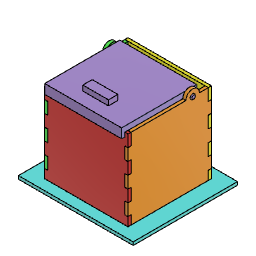
box (Autodesk Fusion 360 design; units mm, degrees)
Autodesk Fusion 360 part; units mm, degrees
note: some values were not read from the file. Set by a fixed rule: which sketch regions a step uses.
sketch "Sketch2" plane through (0, 0, 0) normal (0, 1, 0) x (1, 0, 0)
  line L0 (0, 0) -> (80, 0)
  line L1 (80, 0) -> (80, -80)
  line L2 (80, -80) -> (0, -80)
  line L3 (0, -80) -> (0, 0)
  dimension "d65" = 80
  dimension "d66" = 80
  constraint horizontal L0
  constraint vertical L1
  constraint horizontal L2
  constraint vertical L3
  constraint coincident L0.start L3.end
  measures "d65" distance of L0.start L0.end
  measures "d66" distance of L0.start L2.end
extrude "Extrude1" add sketch "Sketch2" along normal blind 3 makes body 1 in component "Front"
sketch "Sketch1" plane through (0, 0, 0) normal (0, -1, 0) x (1, 0, 0) in component "Front"
  line L0 (80, 80) -> (0, 80)
  line L1 (0, 80) -> (0, 0)
  line L2 (0, 0) -> (80, 0)
  line L3 (80, 0) -> (80, 80)
  line L4 (7.2727, 0) -> (14.5455, 0)
  line L5 (14.5455, 0) -> (14.5455, 3)
  line L6 (14.5455, 3) -> (7.2727, 3)
  line L7 (7.2727, 3) -> (7.2727, 0)
  dimension "d69" = 7.2727
  dimension "d70" = 7.2727
  dimension "d71" = 3
  constraint horizontal L4
  constraint vertical L5
  constraint horizontal L6
  constraint vertical L7
  constraint coincident L2 L4.start
  measures "d69" distance of L5.end L6.end
  measures "d70" distance of L1 L7
  measures "d71" distance of L4 L6
extrude "Extrude2" cut sketch "Sketch1" against normal blind 3 contours L2 L4 L5 L6 L7 bodies 1 in component "Front"
pattern_linear "R-Pattern1" count 5 spacing 14.5455 along (1, 0, 0) of "Extrude2" in component "Front"
sketch "Sketch2 (2)" plane through (80, 0, 0) normal (1, 0, 0) x (0, 1, 0) in component "Front"
  line L0 (0, 80) -> (0, 0)
  line L1 (0, 0) -> (3, 0)
  line L2 (3, 0) -> (3, 80)
  line L3 (3, 80) -> (0, 80)
  line L4 (0, 22.8571) -> (3, 22.8571)
  line L5 (3, 22.8571) -> (3, 11.4286)
  line L6 (3, 11.4286) -> (0, 11.4286)
  line L7 (0, 11.4286) -> (0, 22.8571)
  dimension "d78" = 11.4286
  dimension "d79" = 11.4286
  constraint horizontal L4
  constraint vertical L5
  constraint horizontal L6
  constraint vertical L7
  constraint coincident L2 L5.end
  constraint coincident L0 L4.start
  measures "d78" distance of L4.end L5.end
  measures "d79" distance of L1.end L5.end
extrude "Extrude3" cut sketch "Sketch2 (2)" against normal blind 3 contours L0 L2 L4 L5 L6 L7 bodies 1 in component "Front"
pattern_linear "R-Pattern2" count 3 spacing 22.8571 along (0, 0, 1) of "Extrude3" in component "Front"
ref_plane "WorkPlane1" through (40, 1.5, 74.2857) normal (1, 0, 0) x (0, 0, -1) in component "Front"
mirror "Mirror1" about plane through (40, 1.5, 74.2857) normal (1, 0, 0) of "Extrude3", "R-Pattern2" in component "Front"
sketch "Sketch1 (2)" plane through (80, 0, 0) normal (1, 0, 0) x (0, 1, 0) in component "Right"
  line L0 (3, 11.4286) -> (0, 11.4286)
  line L1 (0, 11.4286) -> (0, 0)
  line L2 (0, 0) -> (3, 0)
  line L3 (3, 0) -> (3, 11.4286)
  line L4 (0, 0) -> (80, 0)
  line L5 (80, 0) -> (80, 80)
  line L6 (80, 80) -> (0, 80)
  line L7 (0, 80) -> (0, 0)
  dimension "d87" = 80
  dimension "d88" = 80
  constraint horizontal L4
  constraint vertical L5
  constraint horizontal L6
  constraint vertical L7
  constraint coincident L1.end L2.start
  measures "d87" distance of L4.end L5.end
  measures "d88" distance of L5.end L6.end
extrude "Extrude1'" add sketch "Sketch1 (2)" against normal blind 3 separate body contours L0 L3 L4 L5 L6 L7 makes body 2 in component "Right"
sketch "Sketch2 (3)" plane through (80, 0, 0) normal (1, 0, 0) x (0, 1, 0) in component "Right"
  line L0 (0, 80) -> (0, 11.4286)
  line L1 (3, 0) -> (80, 0)
  line L2 (80, 0) -> (80, 80)
  line L3 (80, 80) -> (0, 80)
  line L4 (11.4286, 0) -> (22.8571, 0)
  line L5 (22.8571, 0) -> (22.8571, 3)
  line L6 (22.8571, 3) -> (11.4286, 3)
  line L7 (11.4286, 3) -> (11.4286, 0)
  line L8 (0, 11.4286) -> (3, 11.4286)
  line L9 (3, 11.4286) -> (3, 0)
  dimension "d91" = 11.4286
  dimension "d92" = 11.4286
  dimension "d93" = 3
  constraint horizontal L4
  constraint vertical L5
  constraint horizontal L6
  constraint vertical L7
  constraint coincident L1 L4.start
  measures "d91" distance of L5.end L6.end
  measures "d92" distance of L0 L6.end
  measures "d93" distance of L4.end L5.end
extrude "Extrude2'" cut sketch "Sketch2 (3)" against normal blind 3 contours L1 L4 L5 L6 L7 bodies 2 in component "Right"
pattern_linear "R-Pattern1'" count 3 spacing 22.8571 along (0, 1, 0) of "Extrude2'" in component "Right"
ref_plane "WorkPlane1" through (40, 40, 40) normal (0, -1, 0) x (-1, 0, 0)
mirror "MirrorComponent1" about plane through (0, 0, 0) normal (0, 0, 1) of bodies 1 makes body 3 in component "Front(Mirror)"
ref_plane "WorkPlane2" through (40, 1.5, 74.2857) normal (-1, 0, 0) x (0, 0, 1)
combine "Combine1" operation cut target body 2 tool bodies 3 1 body 3 seen with x (1, 0, 0) y (0, -1, 0) z (0, 0, -1) at (0, 80, 0) keep tools in component "Right"
sketch "Sketch3" plane through (80, 0, 0) normal (1, 0, 0) x (0, 1, 0) in component "Right"
  line L0 (3, 11.4286) -> (3, 0)
  line L1 (3, 0) -> (11.4286, 0)
  line L2 (11.4286, 0) -> (11.4286, 3)
  line L3 (11.4286, 3) -> (22.8571, 3)
  line L4 (22.8571, 3) -> (22.8571, 0)
  line L5 (22.8571, 0) -> (34.2857, 0)
  line L6 (34.2857, 0) -> (34.2857, 3)
  line L7 (34.2857, 3) -> (45.7143, 3)
  line L8 (45.7143, 3) -> (45.7143, 0)
  line L9 (45.7143, 0) -> (57.1429, 0)
  line L10 (57.1429, 0) -> (57.1429, 3)
  line L11 (57.1429, 3) -> (68.5714, 3)
  line L12 (68.5714, 3) -> (68.5714, 0)
  line L13 (68.5714, 0) -> (77, 0)
  line L14 (77, 0) -> (77, 11.4286)
  line L15 (77, 11.4286) -> (80, 11.4286)
  line L16 (80, 11.4286) -> (80, 22.8571)
  line L17 (80, 22.8571) -> (77, 22.8571)
  line L18 (77, 22.8571) -> (77, 34.2857)
  line L19 (77, 34.2857) -> (80, 34.2857)
  line L20 (80, 34.2857) -> (80, 45.7143)
  line L21 (80, 45.7143) -> (77, 45.7143)
  line L22 (77, 45.7143) -> (77, 57.1429)
  line L23 (77, 57.1429) -> (80, 57.1429)
  line L24 (80, 57.1429) -> (80, 68.5714)
  line L25 (80, 68.5714) -> (77, 68.5714)
  line L26 (77, 68.5714) -> (77, 80)
  line L27 (77, 80) -> (3, 80)
  line L28 (3, 80) -> (3, 68.5714)
  line L29 (3, 68.5714) -> (0, 68.5714)
  line L30 (0, 68.5714) -> (0, 57.1429)
  line L31 (0, 57.1429) -> (3, 57.1429)
  line L32 (3, 57.1429) -> (3, 45.7143)
  line L33 (3, 45.7143) -> (0, 45.7143)
  line L34 (0, 45.7143) -> (0, 34.2857)
  line L35 (0, 34.2857) -> (3, 34.2857)
  line L36 (3, 34.2857) -> (3, 22.8571)
  line L37 (3, 22.8571) -> (0, 22.8571)
  line L38 (0, 22.8571) -> (0, 11.4286)
  line L39 (0, 11.4286) -> (3, 11.4286)
  circle A0 centre (62, 80) radius 2.5
  circle A1 centre (62, 80) radius 6.5
  dimension "d107" = 4
  dimension "d108" = 15
  dimension "d109" = 5
  constraint coincident L27 A0.centre
  constraint concentric A0 A1
  measures "d107" distance of A0 A1
  measures "d108" distance of L26.end A0.centre
  measures "d109" diameter of A0
extrude "Extrude3'" add sketch "Sketch3" against normal blind 3 contours L27 A0 A1 | L27 A0 picked at (56.9631, 81.0858) picked at (62.5196, 81.3747) bodies 2 in component "Right"
sketch "Sketch3 (2)" plane through (0, 0, 0) normal (0, 0, -1) x (1, 0, 0)
  line L0 (7.2727, -3) -> (7.2727, 0)
  line L1 (7.2727, 0) -> (0, 0)
  line L2 (0, 0) -> (0, -3)
  line L3 (0, -3) -> (7.2727, -3)
  line L4 (-15, 10) -> (95, 10)
  line L5 (95, 10) -> (95, -90)
  line L6 (95, -90) -> (-15, -90)
  line L7 (-15, -90) -> (-15, 10)
  line L8 (0, -80) -> (7.2727, -80)
  line L9 (80, -80) -> (80, -77)
  line L10 (0, -80) -> (0, -77)
  dimension "d115" = 10
  dimension "d116" = 10
  dimension "d117" = 15
  dimension "d118" = 15
  constraint horizontal L4
  constraint vertical L5
  constraint horizontal L6
  constraint vertical L7
  measures "d115" distance of L1 L4
  measures "d116" distance of L6 L8
  measures "d117" distance of L5 L9
  measures "d118" distance of L7 L10
extrude "Extrude1''" add sketch "Sketch3 (2)" against normal blind 3 separate body contours L0 L1 L2 L3 | L4 L5 L6 L7 makes body 4 in component "Bottom"
sketch "Sketch3 (3)" plane through (0, 0, 0) normal (0, -1, 0) x (1, 0, 0) in component "Front"
  line L0 (3, 57.1429) -> (0, 57.1429)
  line L1 (0, 57.1429) -> (0, 45.7143)
  line L2 (0, 45.7143) -> (3, 45.7143)
  line L3 (3, 45.7143) -> (3, 34.2857)
  line L4 (3, 34.2857) -> (0, 34.2857)
  line L5 (0, 34.2857) -> (0, 22.8571)
  line L6 (0, 22.8571) -> (3, 22.8571)
  line L7 (3, 22.8571) -> (3, 11.4286)
  line L8 (3, 11.4286) -> (0, 11.4286)
  line L9 (0, 11.4286) -> (0, 0)
  line L10 (0, 0) -> (7.2727, 0)
  line L11 (7.2727, 0) -> (7.2727, 3)
  line L12 (7.2727, 3) -> (14.5455, 3)
  line L13 (14.5455, 3) -> (14.5455, 0)
  line L14 (14.5455, 0) -> (21.8182, 0)
  line L15 (21.8182, 0) -> (21.8182, 3)
  line L16 (21.8182, 3) -> (29.0909, 3)
  line L17 (29.0909, 3) -> (29.0909, 0)
  line L18 (29.0909, 0) -> (36.3636, 0)
  line L19 (36.3636, 0) -> (36.3636, 3)
  line L20 (36.3636, 3) -> (43.6364, 3)
  line L21 (43.6364, 3) -> (43.6364, 0)
  line L22 (43.6364, 0) -> (50.9091, 0)
  line L23 (50.9091, 0) -> (50.9091, 3)
  line L24 (50.9091, 3) -> (58.1818, 3)
  line L25 (58.1818, 3) -> (58.1818, 0)
  line L26 (58.1818, 0) -> (65.4545, 0)
  line L27 (65.4545, 0) -> (65.4545, 3)
  line L28 (65.4545, 3) -> (72.7273, 3)
  line L29 (72.7273, 3) -> (72.7273, 0)
  line L30 (72.7273, 0) -> (80, 0)
  line L31 (80, 0) -> (80, 11.4286)
  line L32 (80, 11.4286) -> (77, 11.4286)
  line L33 (77, 11.4286) -> (77, 22.8571)
  line L34 (77, 22.8571) -> (80, 22.8571)
  line L35 (80, 22.8571) -> (80, 34.2857)
  line L36 (80, 34.2857) -> (77, 34.2857)
  line L37 (77, 34.2857) -> (77, 45.7143)
  line L38 (77, 45.7143) -> (80, 45.7143)
  line L39 (80, 45.7143) -> (80, 57.1429)
  line L40 (80, 57.1429) -> (77, 57.1429)
  line L41 (77, 57.1429) -> (77, 68.5714)
  line L42 (77, 68.5714) -> (80, 68.5714)
  line L43 (80, 68.5714) -> (80, 80)
  line L44 (80, 80) -> (0, 80)
  line L45 (0, 80) -> (0, 68.5714)
  line L46 (0, 68.5714) -> (3, 68.5714)
  line L47 (3, 68.5714) -> (3, 57.1429)
  line L48 (3.15, 80) -> (76.85, 80)
  line L49 (76.85, 80) -> (76.85, 76)
  line L50 (76.85, 76) -> (3.15, 76)
  line L51 (3.15, 76) -> (3.15, 80)
  dimension "d121" = 73.7
  dimension "d123" = 4
  constraint horizontal L48
  constraint vertical L49
  constraint horizontal L50
  constraint vertical L51
  constraint coincident L44 L48.start
  constraint midpoint L44 L48
  measures "d121" distance of L49.end L50.end
  measures "d123" distance of L48.start L50.end
extrude "Extrude4" cut sketch "Sketch3 (3)" against normal blind 3 contours L44 L48 L49 L50 L51 bodies 1 in component "Front"
sketch "Sketch4" plane through (80, 0, 0) normal (1, 0, 0) x (0, 1, 0) in component "Right"
  line L0 (55.5, 80) -> (3, 80)
  line L1 (3, 80) -> (3, 68.5714)
  line L2 (3, 68.5714) -> (0, 68.5714)
  line L3 (0, 68.5714) -> (0, 57.1429)
  line L4 (0, 57.1429) -> (3, 57.1429)
  line L5 (3, 57.1429) -> (3, 45.7143)
  line L6 (3, 45.7143) -> (0, 45.7143)
  line L7 (0, 45.7143) -> (0, 34.2857)
  line L8 (0, 34.2857) -> (3, 34.2857)
  line L9 (3, 34.2857) -> (3, 22.8571)
  line L10 (3, 22.8571) -> (0, 22.8571)
  line L11 (0, 22.8571) -> (0, 11.4286)
  line L12 (0, 11.4286) -> (3, 11.4286)
  line L13 (3, 0) -> (11.4286, 0)
  line L14 (11.4286, 0) -> (11.4286, 3)
  line L15 (11.4286, 3) -> (22.8571, 3)
  line L16 (22.8571, 3) -> (22.8571, 0)
  line L17 (22.8571, 0) -> (34.2857, 0)
  line L18 (34.2857, 0) -> (34.2857, 3)
  line L19 (34.2857, 3) -> (45.7143, 3)
  line L20 (45.7143, 3) -> (45.7143, 0)
  line L21 (45.7143, 0) -> (57.1429, 0)
  line L22 (57.1429, 0) -> (57.1429, 3)
  line L23 (57.1429, 3) -> (68.5714, 3)
  line L24 (68.5714, 3) -> (68.5714, 0)
  line L25 (68.5714, 0) -> (77, 0)
  line L26 (77, 0) -> (77, 11.4286)
  line L27 (77, 11.4286) -> (80, 11.4286)
  line L28 (80, 11.4286) -> (80, 22.8571)
  line L29 (80, 22.8571) -> (77, 22.8571)
  line L30 (77, 22.8571) -> (77, 34.2857)
  line L31 (77, 34.2857) -> (80, 34.2857)
  line L32 (80, 34.2857) -> (80, 45.7143)
  line L33 (80, 45.7143) -> (77, 45.7143)
  line L34 (77, 45.7143) -> (77, 57.1429)
  line L35 (77, 57.1429) -> (80, 57.1429)
  line L36 (80, 57.1429) -> (80, 68.5714)
  line L37 (80, 68.5714) -> (77, 68.5714)
  line L38 (77, 68.5714) -> (77, 80)
  line L39 (77, 80) -> (68.5, 80)
  arc A0 (68.5, 80) -> (55.5, 80) centre (62, 80) ccw
  circle A1 centre (62, 80) radius 2.5
  line L40 (3, 11.4286) -> (3, 0)
  dimension "d127" = 5
  constraint concentric A0 A1
  measures "d127" diameter of A1
extrude "Extrude4'" cut sketch "Sketch4" against normal blind 3 contours A1 bodies 2 in component "Right"
mirror "MirrorComponent4" about plane through (0, 0, 0) normal (0, 0, 1) of bodies 2 makes body 5 in component "Right(Mirror)"
combine "Combine2" operation cut target body 4 tool bodies 5 3 2 1 body 5 seen with x (-1, 0, 0) y (0, 1, 0) z (0, 0, -1) at (80, 0, 0) body 3 seen with x (1, 0, 0) y (0, -1, 0) z (0, 0, -1) at (0, 80, 0) keep tools in component "Bottom"
ref_plane "WorkPlane1" through (40, 69, 40) normal (0, -1, 0) x (0, 0, 1) in component "Cover"
sketch "Sketch1 (3)" plane through (40, 69, 40) normal (0, -1, 0) x (1, 0, 0) in component "Cover"
  line L0 (-36.85, 45) -> (36.85, 45)
  line L1 (36.85, 45) -> (36.85, 36)
  line L2 (36.85, 36) -> (-36.85, 36)
  line L3 (-36.85, 36) -> (-36.85, 45)
  line L4 (36.85, 36) -> (-36.85, 36)
  line L5 (0, 0) -> (0, 90) construction
  dimension "d131" = 73.7
  dimension "d132" = 9
  constraint horizontal L0
  constraint vertical L1
  constraint horizontal L2
  constraint vertical L3
  constraint collinear L2 L4
  constraint coincident L5.start origin
  constraint perpendicular L0 L5
  constraint midpoint L0 L5
  measures "d131" distance of L0.start L0.end
  measures "d132" distance of L0.end L1.end
extrude "Extrude1'''" add sketch "Sketch1 (3)" along normal blind 72 separate body makes body 6 in component "Cover"
sketch "Sketch2 (4)" plane through (0, 0, 85) normal (0, 0, 1) x (-1, 0, 0) in component "Cover"
  line L0 (-76.85, -69) -> (-3.15, -69)
  line L1 (-3.15, -69) -> (-3.15, 3)
  line L2 (-3.15, 3) -> (-76.85, 3)
  line L3 (-76.85, 3) -> (-76.85, -69)
  line L4 (-27.7167, -9) -> (-52.2833, -9)
  line L5 (-52.2833, -9) -> (-52.2833, -18)
  line L6 (-52.2833, -18) -> (-27.7167, -18)
  line L7 (-27.7167, -18) -> (-27.7167, -9)
  dimension "d136" = 24.5667
  dimension "d137" = 24.5667
  dimension "d138" = 12
  dimension "d139" = 9
  constraint horizontal L4
  constraint vertical L5
  constraint horizontal L6
  constraint vertical L7
  measures "d136" distance of L1 L7
  measures "d137" distance of L3 L5
  measures "d138" distance of L2 L4
  measures "d139" distance of L4.start L6.end
extrude "Extrude2''" add sketch "Sketch2 (4)" along normal blind 5 contours L4 L5 L6 L7 bodies 6 in component "Cover"
sketch "Sketch4 (2)" plane through (76.85, 0, 0) normal (1, 0, 0) x (0, 1, 0)
  line L0 (69, 76) -> (69, 85)
  line L1 (69, 85) -> (-3, 85)
  line L2 (-3, 85) -> (-3, 76)
  line L3 (-3, 76) -> (69, 76)
sketch "Sketch3 (4)" plane through (76.85, 0, 0) normal (1, 0, 0) x (0, 1, 0) in component "Cover"
  line L0 (0, 80) -> (77, 80) construction
  circle A0 centre (62, 80) radius 1.6667
  dimension "d142" = 80
  dimension "d143" = 3.3333
  dimension "d149" = 15
  dimension "d150" = 77
  constraint horizontal L0
  constraint coincident L0 A0.centre
  constraint vertical L0.start origin
  measures "d142" distance of origin L0
  measures "d143" diameter of A0
  measures "d149" distance of L0.end A0.centre
  measures "d150" distance of L0.start L0.end
extrude "Extrude3''" add sketch "Sketch3 (4)" along normal blind 4 bodies 6 in component "Cover"
ref_plane "WorkPlane2" through (40, 33, 80.5) normal (-1, 0, 0) x (0, 0, -1) in component "Cover"
mirror "Mirror1'" about plane through (40, 33, 80.5) normal (-1, 0, 0) of "Extrude3''" in component "Cover"
component "Front" placed x (1, 0, 0) y (0, 1, 0) z (0, 0, 1) at (0, 0, 0)
component "Right" placed x (1, 0, 0) y (0, 1, 0) z (0, 0, 1) at (0, 0, 0)
component "Bottom" placed x (1, 0, 0) y (0, 1, 0) z (0, 0, 1) at (0, 0, 0)
component "Cover" placed x (1, 0, 0) y (0, 1, 0) z (0, 0, 1) at (0, 0, 0)
component "Front(Mirror)" placed x (1, 0, 0) y (0, -1, 0) z (0, 0, -1) at (0, 80, 0)
component "Right(Mirror)" placed x (-1, 0, 0) y (0, 1, 0) z (0, 0, -1) at (80, 0, 0)
equation "thickness = 3 mm" comment "wood thickness"
equation "length = 80 mm" comment "box lenght"
equation "width = 80 mm" comment "box width"
equation "height = 80 mm" comment "box height"
equation "nltabs = 5" comment "number of tabs on length"
equation "nwtabs = 3" comment "number of tabs on width"
equation "nhtabs = 3" comment "number of tabs on height"
equation "ltabs = length / ( nltabs * 2 + 1 )" comment "length of tabs"
equation "wtabs = width / ( nwtabs * 2 + 1 )" comment "width of tabs"
equation "htabs = height / ( nhtabs * 2 + 1 )" comment "height of tabs"
equation "hole = 5 mm"
equation "d65 = length"
equation "d66 = height"
equation "d67 = thickness"
equation "d69 = ltabs"
equation "d70 = d69"
equation "d71 = thickness"
equation "d72 = -thickness"
equation "d74 = nltabs"
equation "d76 = -( length - ltabs * 3 )"
equation "d78 = htabs"
equation "d79 = d78"
equation "d80 = -thickness"
equation "d82 = nhtabs"
equation "d84 = -( height - htabs * 3 )"
equation "d87 = height"
equation "d88 = width"
equation "d89 = -thickness"
equation "d91 = wtabs"
equation "d92 = d91"
equation "d93 = thickness"
equation "d94 = -thickness"
equation "d98 = -( width - wtabs * 3 )"
equation "d109 = hole"
equation "d110 = -thickness"
equation "d116 = d115"
equation "d118 = d117"
equation "d119 = -thickness"
equation "d121 = coverlength"
equation "coverlength = length - thickness * 2 - 0.3 mm" comment "cover length"
equation "d123 = coverthickness"
equation "coverthickness = 4 mm" comment "cover thickness"
equation "d125 = -thickness"
equation "d127 = hole"
equation "d128 = -thickness"
equation "d131 = coverlength"
equation "d132 = coverthickness + hole"
equation "coverwidth = width - 8 mm" comment "cover width"
equation "d134 = coverwidth"
equation "d136 = coverlength / 3"
equation "d137 = d136"
equation "d142 = height"
equation "d143 = hole / 1.5"
equation "d150 = width - thickness"
